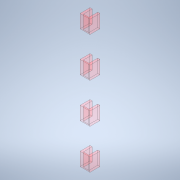
# Autodesk Inventor part: RedLights-ver-1-1111-2021
Saved by Autodesk Inventor 2021 (Build 250183000, 183)
## iProperties
Created: 2021-03-03
Part Number: RedLights-ver-1-1111-2021
Material: Generic
Document SubType Name: Modeling
Designer: CMurray
Density: 1 g/cm^3
Appearance: Polycarbonate - Clear
Author: CMurray
Autodesk Inventor part; units mm, degrees
sketch "Sketch2" plane through (0, 0, 0) normal (1, 0, 0) x (0, 1, 0)
  line L0 (0, 0) -> (0, -1828.8)
  line L1 (0, 0) -> (2133.6, 0)
  line L2 (2133.6, 0) -> (0, -1828.8)
  line L3 (0, 0) -> (152.4, 0)
  line L4 (152.4, 0) -> (685.8, 0)
  line L5 (2133.6, 0) -> (1981.2, 0)
  line L6 (1981.2, 0) -> (1854.2, 0)
  line L7 (1854.2, 0) -> (1549.4, 0)
  line L8 (1549.4, 0) -> (1422.4, 0)
  line L9 (1422.4, 0) -> (1117.6, 0)
  line L10 (1117.6, 0) -> (990.6, 0)
  line L11 (990.6, 0) -> (685.8, 0)
  line L12 (685.8, 0) -> (558.8, 0)
  line L13 (558.8, 0) -> (254, 0)
  line L14 (0, 0) -> (304.8, 0)
  line L15 (304.8, 0) -> (457.2, 0)
  line L16 (457.2, 0) -> (762, 0)
  line L17 (762, 0) -> (914.4, 0)
  line L18 (914.4, 0) -> (1219.2, 0)
  line L19 (1219.2, 0) -> (1371.6, 0)
  line L20 (1371.6, 0) -> (1676.4, 0)
  line L21 (1676.4, 0) -> (1828.8, 0)
  line L22 (304.8, 0) -> (304.8, -101.6)
  line L23 (457.2, 0) -> (457.2, -101.6)
  line L24 (762, 0) -> (762, -101.6)
  line L25 (914.4, 0) -> (914.4, -101.6)
  line L26 (1219.2, 0) -> (1219.2, -101.6)
  line L27 (1371.6, 0) -> (1371.6, -101.6)
  line L28 (1676.4, 0) -> (1676.4, -101.6)
  line L29 (1828.8, 0) -> (1828.8, -101.6)
  line L30 (1828.8, -101.6) -> (1676.4, -101.6)
  line L31 (1371.6, -101.6) -> (1219.2, -101.6)
  line L32 (914.4, -101.6) -> (762, -101.6)
  line L33 (457.2, -101.6) -> (304.8, -101.6)
  point P0 (304.8, -1567.5429)
  point P1 (457.2, -1436.9143)
  point P2 (762, -1175.6571)
  point P3 (914.4, -1045.0286)
  point P4 (1219.2, -783.7714)
  point P5 (1371.6, -653.1429)
  point P6 (1676.4, -391.8857)
  point P7 (1828.8, -261.2571)
  dimension "d1" = 1828.8
  dimension "d3" = 152.4
  dimension "d5" = 152.4
  dimension "d14" = 304.8
  dimension "d15" = 152.4
  dimension "d16" = 304.8
  dimension "d17" = 152.4
  dimension "d18" = 304.8
  dimension "d19" = 152.4
  dimension "d20" = 304.8
  dimension "d21" = 152.4
  dimension "d24" = 2133.6
  dimension "d27" = 101.6
  dimension "d28" = 101.6
  dimension "d29" = 101.6
  constraints: 64 end point, 12 point on line, 7 parallel, 3 perpendicular, 2 vertical, 1 collinear, 22 other
  measures "d1" distance of L0.start L0.end
  measures "d3" distance of L0.start L3.end
  measures "d5" distance of L5.start L5.end
  measures "d14" distance of L0.start L14.end
  measures "d15" distance of L14.end L15.end
  measures "d16" distance of L15.end L16.end
  measures "d17" distance of L16.end L17.end
  measures "d18" distance of L17.end L18.end
  measures "d19" distance of L18.end L19.end
  measures "d20" distance of L19.end L20.end
  measures "d21" distance of L20.end L21.end
  measures "d24" distance from line of L0 L5.start
  measures "d27" distance of the line from the sketch origin of L30
  measures "d28" distance of the line from the sketch origin of L31
  measures "d29" distance between parallel lines of L33 L15
extrude "Extrusion1" add sketch "Sketch2" along normal blind 25.4 contours L1 L23 L33 L22 | L29 L30 L28 L1 | L1 L25 L32 L24 | L27 L31 L26 L1
ref_plane "Work Plane3" through (12.7, 914.4, 0) normal (0, 0, 1) x (1, 0, 0)
sketch "Sketch5" plane through (0, 762, 0) normal (0, 0, 1) x (1, 0, 0)
  line L0 (25.4, -304.8) -> (25.4, -457.2) projected
  line L1 (0, -304.8) -> (25.4, -304.8) projected
  line L2 (25.4, -457.2) -> (0, -457.2)
  line L3 (0, -457.2) -> (0, -304.8)
  line L4 (0, -304.8) -> (25.4, -304.8)
  line L5 (25.4, -304.8) -> (25.4, -457.2)
  line L6 (25.4, 152.4) -> (25.4, 0) projected
  line L7 (0, 152.4) -> (25.4, 152.4) projected
  line L8 (25.4, 0) -> (0, 0)
  line L9 (0, 0) -> (0, 152.4)
  line L10 (0, 152.4) -> (25.4, 152.4)
  line L11 (25.4, 152.4) -> (25.4, 0)
  line L12 (25.4, 609.6) -> (25.4, 457.2) projected
  line L13 (0, 609.6) -> (0, 457.2) projected
  line L14 (25.4, 457.2) -> (0, 457.2)
  line L15 (0, 457.2) -> (0, 609.6)
  line L16 (0, 609.6) -> (25.4, 609.6)
  line L17 (25.4, 609.6) -> (25.4, 457.2)
  line L18 (25.4, 1066.8) -> (25.4, 914.4) projected
  line L19 (0, 1066.8) -> (0, 914.4) projected
  line L20 (25.4, 914.4) -> (0, 914.4)
  line L21 (0, 914.4) -> (0, 1066.8)
  line L22 (0, 1066.8) -> (25.4, 1066.8)
  line L23 (25.4, 1066.8) -> (25.4, 914.4)
  point P0 (0, -762)
  constraints: 32 end point, 8 parallel, 4 horizontal, 4 perpendicular
extrude "Extrusion3" add sketch "Sketch5" along normal blind 12.7
ref_plane "Work Plane5" through (0, 0, 0) normal (-1, 0, 0) x (0, 0, 1)
ref_plane "Work Plane4" through (12.7, 0, 0) normal (-1, 0, 0) x (0, 0, 1)
sketch "Sketch6" plane through (0, 0, 0) normal (-1, 0, 0) x (0, 0, 1)
  line L0 (-101.6, 304.8) -> (12.7, 304.8) projected
  line L1 (-101.6, 457.2) -> (12.7, 457.2) projected
  line L2 (12.7, 304.8) -> (0, 304.8)
  line L3 (0, 304.8) -> (0, 457.2)
  line L4 (0, 457.2) -> (12.7, 457.2)
  line L5 (12.7, 457.2) -> (12.7, 304.8)
  line L6 (-101.6, 762) -> (12.7, 762) projected
  line L7 (-101.6, 914.4) -> (12.7, 914.4) projected
  line L8 (12.7, 762) -> (0, 762)
  line L9 (0, 762) -> (0, 914.4)
  line L10 (0, 914.4) -> (12.7, 914.4)
  line L11 (12.7, 914.4) -> (12.7, 762)
  line L12 (12.7, 1371.6) -> (12.7, 1219.2) projected
  line L13 (12.7, 1219.2) -> (0, 1219.2)
  line L14 (0, 1219.2) -> (0, 1371.6)
  line L15 (0, 1371.6) -> (12.7, 1371.6)
  line L16 (12.7, 1371.6) -> (12.7, 1219.2)
  line L17 (-101.6, 1676.4) -> (12.7, 1676.4) projected
  line L18 (-101.6, 1828.8) -> (12.7, 1828.8) projected
  line L19 (12.7, 1676.4) -> (0, 1676.4)
  line L20 (0, 1676.4) -> (0, 1828.8)
  line L21 (0, 1828.8) -> (12.7, 1828.8)
  line L22 (12.7, 1828.8) -> (12.7, 1676.4)
  point P0 (0, 0)
  point P1 (0, 304.8)
  dimension "d33" = 12.7
  constraints: 32 end point, 8 parallel, 5 point on line, 4 horizontal, 4 perpendicular
  measures "d33" distance between parallel lines of L5 L3
extrude "Extrusion4" add sketch "Sketch6" along normal blind 88.9
ref_plane "Work Plane6" through (-44.45, 304.8, 0) normal (0, 0, -1) x (-1, 0, 0)
sketch "Sketch7" plane through (0, 762, 0) normal (0, 0, -1) x (-1, 0, 0)
  line L0 (0, 914.4) -> (88.9, 914.4) projected
  line L1 (0, 1066.8) -> (88.9, 1066.8) projected
  line L2 (88.9, 914.4) -> (63.5, 914.4)
  line L3 (63.5, 914.4) -> (63.5, 1066.8)
  line L4 (63.5, 1066.8) -> (88.9, 1066.8)
  line L5 (88.9, 1066.8) -> (88.9, 914.4)
  line L6 (0, 457.2) -> (88.9, 457.2) projected
  line L7 (0, 609.6) -> (88.9, 609.6) projected
  line L8 (88.9, 457.2) -> (63.5, 457.2)
  line L9 (63.5, 457.2) -> (63.5, 609.6)
  line L10 (63.5, 609.6) -> (88.9, 609.6)
  line L11 (88.9, 609.6) -> (88.9, 457.2)
  line L12 (88.9, 152.4) -> (88.9, 0) projected
  line L13 (0, 152.4) -> (88.9, 152.4) projected
  line L14 (88.9, 0) -> (63.5, 0)
  line L15 (63.5, 0) -> (63.5, 152.4)
  line L16 (63.5, 152.4) -> (88.9, 152.4)
  line L17 (88.9, 152.4) -> (88.9, 0)
  line L18 (0, -304.8) -> (88.9, -304.8) projected
  line L19 (88.9, -457.2) -> (63.5, -457.2)
  line L20 (63.5, -457.2) -> (63.5, -304.8)
  line L21 (63.5, -304.8) -> (88.9, -304.8)
  line L22 (88.9, -304.8) -> (88.9, -457.2)
  point P0 (0, -762)
  dimension "d36" = 25.4
  constraints: 32 end point, 8 parallel, 6 point on line, 4 horizontal, 4 perpendicular
  measures "d36" distance between parallel lines of L5 L3
extrude "Extrusion5" add sketch "Sketch7" along normal blind 101.6
body "Solid1"
